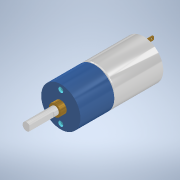
# Autodesk Inventor part: motor_dc_20d_12v
Saved by Autodesk Inventor 2020.2 (Build 242310000, 310)
## iProperties
Created: 2020-02-20
Part Number: motor_dc_20d_12v
Material: Generic
Document SubType Name: Modeling
Designer: Bardo91
Density: 1 g/cm^3
Appearance: Default
Author: Bardo91
Autodesk Inventor part; units mm, degrees
ref_plane "YZ Plane" through (0, 0, 0) normal (1, 0, 0) x (0, 1, 0)
ref_plane "XZ Plane" through (0, 0, 0) normal (0, 1, 0) x (-1, 0, 0)
ref_plane "XY Plane" through (0, 0, 0) normal (0, 0, 1) x (1, 0, 0)
sketch "Sketch1" plane through (0, 0, 0) normal (0, 0, 1) x (1, 0, 0)
  circle A0 centre (0, 0) radius 10
  dimension "d0" = 20
  constraints: 1 centre point, 1 coincident
  measures "d0" diameter of A0
extrude "Extrusion1" add sketch "Sketch1" along normal blind 17.3
sketch "Sketch2" plane through (0, 0, 17.3) normal (0, 0, 1) x (1, 0, 0)
  line L0 (0, 0) -> (0, 7.5)
  circle A0 centre (0, 7.5) radius 1.25
  line L1 (0, 0) -> (0, -7.5)
  circle A1 centre (0, -7.5) radius 1.25
  dimension "d3" = 7.5
  dimension "d4" = 2.5
  dimension "d5" = 7.5
  dimension "d6" = 2.5
  constraints: 4 end point, 2 centre point, 2 coincident, 2 vertical
  measures "d3" distance of L0.start L0.end
  measures "d4" diameter of A0
  measures "d5" distance of L0.start L1.end
  measures "d6" diameter of A1
extrude "Extrusion2" cut sketch "Sketch2" against normal blind 1
sketch "Sketch3" plane through (0, 0, 17.3) normal (0, 0, 1) x (1, 0, 0)
  circle A0 centre (0, 0) radius 3
  dimension "d9" = 6
  constraints: 1 centre point, 1 coincident
  measures "d9" diameter of A0
extrude "Extrusion3" add sketch "Sketch3" along normal blind 3
sketch "Sketch4" plane through (0, 0, 20.3) normal (0, 0, 1) x (1, 0, 0)
  circle A0 centre (0, 0) radius 2
  dimension "d12" = 4
  constraints: 1 centre point, 1 coincident
  measures "d12" diameter of A0
extrude "Extrusion4" add sketch "Sketch4" along normal blind 14.5
sketch "Sketch5" plane through (0, 0, 34.8) normal (0, 0, 1) x (1, 0, 0)
  line L0 (0, 0) -> (2, 0)
  line L1 (2, 0) -> (1.5, 0)
  circle A0 centre (0, 0) radius 2
  line L2 (1.5, 0) -> (1.5, 1.3229)
  line L3 (1.5, 0) -> (1.5, -1.3229)
  circle A1 centre (0, 0) radius 2 projected
  dimension "d17" = 4
  dimension "d15" = 2
  dimension "d16" = 0.5
  constraints: 8 end point, 2 point on line, 1 coincident, 1 horizontal, 1 point on circle, 1 vertical, 3 other
  measures "d15" distance of L0.start L0.end
  measures "d16" distance of L0.end L1.end
extrude "Extrusion5" cut sketch "Sketch5" against normal blind 12.2 contours L2 A0 L0 | L0 A0 L3
sketch "Sketch7" plane through (0, 0, 0) normal (1, 0, 0) x (0, 1, 0)
  line L0 (10, 0) -> (-10, 0) projected
  line L1 (0, 0) -> (9, 0)
  line L2 (10, -1) -> (10, -25)
  line L3 (10, -25) -> (0, -25)
  line L4 (0, -25) -> (0, 0)
  arc A0 (10, -1) -> (9, 0) centre (9, -1) ccw
  line L5 (0, -25) -> (0, -28)
  line L6 (0, -28) -> (3, -28)
  line L7 (3, -28) -> (4.7321, -25)
  dimension "d20" = 10
  dimension "d21" = 25
  dimension "d22" = 1
  dimension "d23" = 3
  dimension "d24" = 3
  dimension "d25" = 120
  constraints: 14 end point, 4 perpendicular, 3 point on line, 2 point on circle, 2 tangent, 1 centre point, 1 collinear, 1 vertical
  measures "d20" distance of L1.start L0.start
  measures "d21" distance of L0.start L2.end
  measures "d22" radius of A0
  measures "d23" distance of L3.end L5.end
  measures "d24" distance of L5.end L6.end
  measures "d25" angle of L7 L6
revolve "Revolution1" add sketch "Sketch7" angle 360 about axis through (0, 0, -25) along (0, 0, 1)
sketch "Sketch8" plane through (0, 0, 0) normal (1, 0, 0) x (0, 1, 0)
  line L0 (-4.7321, -25) -> (4.7321, -25) projected
  line L1 (0, -25) -> (8, -25)
  line L2 (8, -25) -> (8, -29.5)
  line L3 (7.5, -30) -> (6.5, -30)
  line L4 (6, -29.5) -> (6, -25)
  arc A0 (7.5, -30) -> (8, -29.5) centre (7.5, -29.5) ccw
  arc A1 (6, -29.5) -> (6.5, -30) centre (6.5, -29.5) ccw
  line L5 (-10, -25) -> (10, -25) projected
  line L6 (7, -25) -> (7, -29)
  circle A2 centre (7, -29) radius 0.5
  line L7 (0, -25) -> (0, -32)
  line L8 (0, -25) -> (-8, -25)
  line L9 (-8, -25) -> (-8, -29.5)
  line L10 (-7.5, -30) -> (-6.5, -30)
  line L11 (-6, -29.5) -> (-6, -25)
  arc A3 (-8, -29.5) -> (-7.5, -30) centre (-7.5, -29.5) ccw
  arc A4 (-6.5, -30) -> (-6, -29.5) centre (-6.5, -29.5) ccw
  line L12 (-7, -25) -> (-7, -29)
  circle A5 centre (-7, -29) radius 0.5
  point P0 (0, 0)
  point P1 (8, -30)
  point P2 (6, -30)
  point P3 (-8, -30)
  point P4 (-6, -30)
  point P5 (-8, -25)
  point P6 (-6, -25)
  dimension "d27" = 8
  dimension "d28" = 5
  dimension "d29" = 2
  dimension "d30" = 0.5
  dimension "d31" = 4
  dimension "d32" = 1
  dimension "d33" = 7
  constraints: 22 end point, 13 symmetric about line, 11 point on line, 8 point on circle, 6 centre point, 5 perpendicular, 4 tangent, 2 coincident, 1 collinear, 1 equal radius, 1 midpoint, 3 other
  measures "d27" distance of L1.start L1.end
  measures "d28" distance of L1.end point (8, -30)
  measures "d29" distance of point (8, -30) point (6, -30)
  measures "d30" radius of A0
  measures "d31" distance of L6.start L6.end
  measures "d32" diameter of A2
  measures "d33" distance of L1.start L7.end
extrude "Extrusion6" add sketch "Sketch8" along normal mid plane 0.5
body "Solid1"
